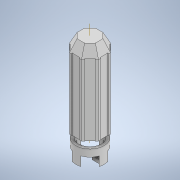
# Autodesk Inventor part: LED base
Saved by Autodesk Inventor 2020 (Build 240168000, 168)
## iProperties
Created: 2019-10-11
Part Number: LED base
Material: Generic
Document SubType Name: Modeling
Designer: cpick
Density: 1 g/cm^3
Appearance: Default
Author: cpick
Autodesk Inventor part; units mm, degrees
ref_plane "YZ Plane" through (0, 0, 0) normal (1, 0, 0) x (0, 1, 0)
ref_plane "XZ Plane" through (0, 0, 0) normal (0, 1, 0) x (-1, 0, 0)
sketch "Sketch1" plane through (0, 0, 0) normal (0, 1, 0) x (-1, 0, 0)
  line L0 (20.5, -8.4914) -> (8.4914, -20.5)
  line L1 (8.4914, -20.5) -> (-8.4914, -20.5)
  line L2 (-8.4914, -20.5) -> (-20.5, -8.4914)
  line L3 (-20.5, -8.4914) -> (-20.5, 8.4914)
  line L4 (-20.5, 8.4914) -> (-8.4914, 20.5)
  line L5 (-8.4914, 20.5) -> (8.4914, 20.5)
  line L6 (8.4914, 20.5) -> (20.5, 8.4914)
  line L7 (20.5, 8.4914) -> (20.5, -8.4914)
  point P0 (0, 0)
  point P1 (0, 0)
  dimension "d0" = 41
  constraints: 16 end point, 1 coincident, 17 other
  measures "d0" distance between parallel lines of L3 L7
extrude "Extrusion1" add sketch "Sketch1" along normal blind 100
ref_plane "Work Plane1" through (0, 115, 0) normal (0, 1, 0) x (1, 0, 0)
sketch "Sketch2" plane through (0, 115, 0) normal (0, 1, 0) x (1, 0, 0)
  line L0 (-13, 5.3848) -> (-5.3848, 13)
  line L1 (-5.3848, 13) -> (5.3848, 13)
  line L2 (5.3848, 13) -> (13, 5.3848)
  line L3 (13, 5.3848) -> (13, -5.3848)
  line L4 (13, -5.3848) -> (5.3848, -13)
  line L5 (5.3848, -13) -> (-5.3848, -13)
  line L6 (-5.3848, -13) -> (-13, -5.3848)
  line L7 (-13, -5.3848) -> (-13, 5.3848)
  point P0 (0, 0)
  point P1 (0, 0)
  dimension "d4" = 26
  constraints: 16 end point, 1 coincident, 17 other
  measures "d4" distance between parallel lines of L3 L7
loft "Loft1" add profiles "Sketch2" section 1 edges at (14.4957, 100, -14.4957) (0, 100, -20.5) (-14.4957, 100, -14.4957) (-20.5, 100, 0) (-14.4957, 100, 14.4957) (0, 100, 20.5) (14.4957, 100, 14.4957) (20.5, 100, 0)
sketch "Sketch3" plane through (0, 0, 0) normal (0, -1, 0) x (1, 0, 0)
  line L0 (21.3077, 5.2499) -> (20, 5.2499)
  line L1 (20, 5.2499) -> (20, -5.2501)
  line L2 (20, -5.2501) -> (21.3077, -5.2501)
  line L3 (21.3077, -5.2501) -> (21.3077, 5.2499)
  line L4 (8.4914, 20.5) -> (20.5, 8.4914) projected
  line L5 (20.5, -8.4914) -> (8.4914, -20.5) projected
  line L6 (20.5, 8.4914) -> (20.5, -8.4914) projected
  point P0 (0, 0)
  dimension "d9" = 10.5
  dimension "d10" = 3.2415
  dimension "d11" = 0.5
  constraints: 8 end point, 2 parallel, 1 horizontal, 1 perpendicular
  measures "d9" distance of L2.end L0.start
  measures "d10" distance from line of L0 L4.end
  measures "d11" distance between parallel lines of L6 L1
extrude "Extrusion2" cut sketch "Sketch3" against normal through all
pattern_circular "Circular Pattern1" count 8 over 360 about axis through (0, 0, 0) along (0, -1, 0) of "Extrusion2"
sketch "Sketch4" plane through (0, 0, 0) normal (0, -1, 0) x (1, 0, 0)
  circle A0 centre (0, 0) radius 20
  circle A1 centre (0, 0) radius 16
  line L0 (-10.4297, 17.8545) -> (-17.8544, 10.4299) projected
  dimension "d28" = 32
  constraints: 2 centre point, 2 coincident, 1 tangent
  measures "d28" diameter of A1
extrude "Extrusion3" add sketch "Sketch4" along normal blind 23 separate body
sketch "Sketch5" plane through (10.4299, 0, 17.8544) normal (0.7071068, 0, 0.7071068) x (0.7071068, 0, -0.7071068)
  line L0 (-4, -10) -> (14.5, -10)
  line L1 (14.5, -10) -> (14.5, -32.8692)
  line L2 (14.5, -32.8692) -> (-4, -32.8692)
  line L3 (-4, -32.8692) -> (-4, -10)
  line L4 (0, 0) -> (0, 100) projected
  line L5 (10.5, 100) -> (10.5, 0) projected
  line L6 (10.5, 0) -> (0, 0) projected
  point P0 (5.2499, 0)
  dimension "d19" = 4
  dimension "d20" = 4
  dimension "d21" = 10
  constraints: 8 end point, 2 parallel, 1 horizontal, 1 perpendicular
  measures "d19" distance between parallel lines of L3 L4
  measures "d20" distance between parallel lines of L1 L5
  measures "d21" distance between parallel lines of L0 L6
extrude "Extrusion4" cut sketch "Sketch5" against normal through all bodies 1 2
sketch "Sketch6" plane through (17.8544, 0, -10.4299) normal (0.7071068, 0, -0.7071068) x (-0.7071068, 0, -0.7071068)
  line L0 (-4, -10) -> (14.5, -10)
  line L1 (14.5, -10) -> (14.5, -24.5783)
  line L2 (14.5, -24.5783) -> (-4, -24.5783)
  line L3 (-4, -24.5783) -> (-4, -10)
  line L4 (0, 0) -> (0, 100) projected
  line L5 (10.5, 100) -> (10.5, 0) projected
  point P0 (5.2499, 0)
  dimension "d24" = 4
  dimension "d25" = 4
  constraints: 8 end point, 2 parallel, 1 horizontal, 1 perpendicular
  measures "d24" distance between parallel lines of L3 L4
  measures "d25" distance between parallel lines of L1 L5
extrude "Extrusion5" cut sketch "Sketch6" against normal through all bodies 1 2
move or copy body "Move Body1" bodies to move or copy 2 copy no translate (0, -10, 0)
sketch "Sketch7" plane through (-19.0794, -33, -5.9981) normal (0, -1, 0) x (0.7071068, 0, -0.7071068)
  line L0 (-3.8052, 8.4823) -> (-8.4824, 8.4823) projected
  arc A0 (-8.4824, 8.4823) -> (0, 0) centre (9.2499, 17.7324) ccw projected
  line L1 (0, 0) -> (0, 4.6772) projected
  arc A1 (-3.8052, 8.4823) -> (0, 4.6772) centre (9.2499, 17.7324) ccw projected
  line L2 (0, 4.6772) -> (0, 0) projected
  arc A2 (-3.8054, 26.9823) -> (-3.8052, 8.4823) centre (9.2499, 17.7324) ccw projected
  line L3 (-3.8052, 8.4823) -> (3.2658, 15.5535)
  line L4 (3.2658, 15.5535) -> (7.071, 11.7483)
  line L5 (7.071, 11.7483) -> (0, 4.6772)
  arc A3 (18.5, 4.6774) -> (22.305, 8.4823) centre (9.2499, 17.7324) ccw projected
  line L6 (9.2499, 17.7324) -> (-2.0639, 29.0461)
  circle A4 centre (9.2499, 17.7324) radius 16 projected
  line L7 (18.4998, 30.7877) -> (11.4288, 23.7166)
  line L8 (11.4288, 23.7166) -> (15.234, 19.9114)
  line L9 (15.234, 19.9114) -> (22.305, 26.9826)
  point P0 (18.4998, 30.7877)
  dimension "d32" = 10
  constraints: 14 end point, 4 symmetric about line, 1 parallel, 1 point on circle
  measures "d32" distance of L0.start L3.end
extrude "Extrusion6" add sketch "Sketch7" against normal blind 5 contours L3 L4 L5 A1 | A4 L9 L8 L7 bodies 2
sketch "Sketch8" plane through (0, -33, 0) normal (0, -1, 0) x (1, 0, 0.0000069)
  line L0 (-15.1014, 0) -> (-7.1014, 0) construction
  line L1 (-13.6014, -1.5) -> (-8.6014, -1.5)
  line L2 (-8.6014, 1.5) -> (-13.6014, 1.5)
  arc A0 (-13.6014, 1.5) -> (-13.6014, -1.5) centre (-13.6014, 0) ccw
  arc A1 (-8.6014, -1.5) -> (-8.6014, 1.5) centre (-8.6014, 0) ccw
  line L3 (0, 0) -> (0, 5.7569)
  line L4 (15.1014, 0) -> (7.1014, 0) construction
  line L5 (13.6014, -1.5) -> (8.6014, -1.5)
  line L6 (8.6014, 1.5) -> (13.6014, 1.5)
  arc A2 (13.6014, -1.5) -> (13.6014, 1.5) centre (13.6014, 0) ccw
  arc A3 (8.6014, 1.5) -> (8.6014, -1.5) centre (8.6014, 0) ccw
  line L7 (-5.7721, -2.6907) -> (-5.7721, 2.6906) projected
  line L8 (-5.7721, 0) -> (-15.667, 0)
  point P0 (-11.1014, 0)
  point P1 (11.1014, 0)
  dimension "d35" = 3
  dimension "d38" = 5
  constraints: 20 end point, 12 point on circle, 9 symmetric about line, 5 point on line, 4 centre point, 4 tangent, 2 horizontal, 2 midpoint, 1 parallel, 1 vertical, 2 other
  measures "d35" diameter of A1
  measures "d38" distance of L2.start L2.end
extrude "Extrusion7" cut sketch "Sketch8" against normal blind 5 bodies 2
body "Solid1"
body "Solid2"
